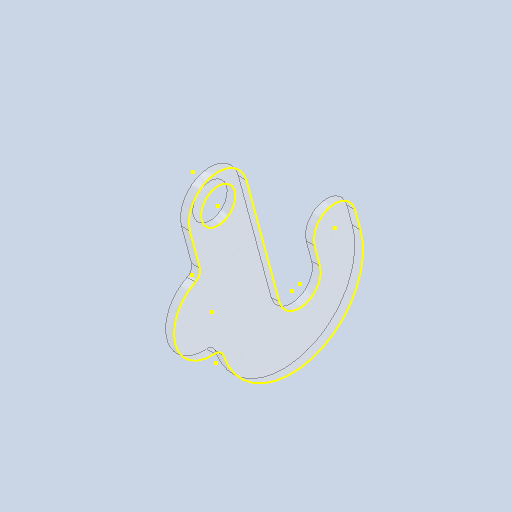
# Autodesk Inventor part: part3
Saved by Autodesk Inventor 2025.2 (Build 292293000, 293)
## iProperties
Created: 2025-02-28
Part Number: part3
Material: アクリル、クリア
Document SubType Name: Modeling
Designer: haruy
Density: 1.19 g/cm^3
Appearance: 透明 - クリア
Author: haruy
Autodesk Inventor part; units mm, degrees
ref_plane "YZ Plane" through (0, 0, 0) normal (1, 0, 0) x (0, 1, 0)
ref_plane "XZ Plane" through (0, 0, 0) normal (0, 1, 0) x (-1, 0, 0)
ref_plane "XY Plane" through (0, 0, 0) normal (0, 0, 1) x (1, 0, 0)
derived "oikon-Sketch-Base.ipt"
sketch "スケッチ1" plane through (100, 0, 0) normal (1, 0, 0) x (0, 1, 0)
  line L0 (0, 0) -> (-50, 0)
  line L1 (-50, 0) -> (-50, -2)
  line L2 (-50, -2) -> (0, -2)
  line L3 (0, -2) -> (0, 0)
  circle A0 centre (-10, -6) radius 4 construction
  circle A1 centre (-10, -6) radius 7
  line L4 (-26, 13) -> (-45, 13)
  line L5 (-45, 13) -> (-45, 2.35)
  line L6 (-45, 2.35) -> (-26, 2.35)
  line L7 (-26, 2.35) -> (-26, 13)
  line L8 (0, 14.6) -> (-50, 14.6)
  line L9 (-50, 14.6) -> (-50, 13)
  line L10 (-50, 13) -> (0, 13)
  line L11 (0, 13) -> (0, 14.6)
  line L12 (0, 36.6) -> (-50, 36.6)
  line L13 (-50, 36.6) -> (-50, 34.6)
  line L14 (-50, 34.6) -> (0, 34.6)
  line L15 (0, 34.6) -> (0, 36.6)
  line L16 (-11.8238, 0.7582) -> (-40.7877, -7.0578)
  arc A2 (-34, 2.35) -> (-32, 2.35) centre (-33, 2.35) ccw
  line L17 (-8.1762, -12.7582) -> (-37.1402, -20.5743)
  line L18 (-40.7877, -7.0578) -> (-37.1402, -20.5743)
  line L19 (-37.1402, -20.5743) -> (-31.9295, -39.8836)
  arc A3 (-37.1402, -20.5743) -> (-34.5348, -30.229) centre (-35.8375, -25.4016) ccw
  line L20 (-34.5348, -30.229) -> (-29.7075, -28.9263)
  line L21 (-29.7075, -28.9263) -> (-28.6397, -32.8834)
  arc A4 (-27.1021, -38.5809) -> (-29.7075, -28.9263) centre (-28.4048, -33.7536) ccw
  line L22 (-27.1021, -38.5809) -> (-31.9295, -39.8836)
  arc A5 (-40.7877, -7.0578) -> (-31.9295, -39.8836) centre (-36.3586, -23.4707) ccw
  line L23 (0, 0) -> (5, 0)
  line L24 (5, 0) -> (5, -2)
  line L25 (5, -2) -> (0, -2)
  line L26 (0, -2) -> (0, 0)
  line L27 (0, 36.6) -> (5, 36.6)
  line L28 (5, 36.6) -> (5, 34.6)
  line L29 (5, 34.6) -> (0, 34.6)
  line L30 (0, 34.6) -> (0, 36.6)
  line L31 (-50, 36.6) -> (-55, 36.6)
  line L32 (-55, 36.6) -> (-55, 34.6)
  line L33 (-55, 34.6) -> (-50, 34.6)
  line L34 (-50, 34.6) -> (-50, 36.6)
  line L35 (-50, 0) -> (-55, 0)
  line L36 (-55, 0) -> (-55, -2)
  line L37 (-55, -2) -> (-50, -2)
  line L38 (-50, -2) -> (-50, 0)
  circle A6 centre (-10, -6) radius 4.1
  arc A7 (-22.4439, -2.1076) -> (-39.8222, -6.7973) centre (-31.133, -4.4525) ccw
  point P0 (-14.1989, 2.35)
  point P1 (-31.9295, -39.8836)
  dimension "d1" = 8.2
  measures "d1" diameter of A6
extrude "押し出し1" add sketch "スケッチ1" along normal blind 2 contours A1 L2 A6 L0 | L0 A1 | A1 L2 L16 L0 | L0 L16 A1 | A1 L2 A6 | A1 L17 L18 L16 L2 | A7 L2 L0 | L0 A7 L6 A2 L7 | A7 L16 L2 | L7 L6 A7 | A3 L19 A5 L18 | L20 A4 L22 L19 | L6 A2 picked at (-34.1225, -4.7033)
fillet "フィレット1" radius 2 2 edges at (101, -22.4439, -2.1076) (101, -39.8222, -6.7973)
sketch "スケッチ2" plane through (102, -37.1402, -20.5743) normal (1, 0, 0) x (0, 0.2605359, -0.9654642)
  arc A0 (-13.9842, -0.7336) -> (20, 0) centre (3, 0) ccw projected
  line L0 (20, 0) -> (20, 5) projected
  arc A1 (20, 5) -> (10, 5) centre (15, 5) ccw projected
  line L1 (10, 5) -> (10, 0) projected
  arc A2 (0, 0) -> (10, 0) centre (5, 0) ccw projected
  line L2 (0, 0) -> (0, 30) projected
  arc A3 (0, 30) -> (-14, 30) centre (-7, 30) ccw projected
  line L3 (-14, 30) -> (-14, 20.8167) projected
  arc A4 (-15.6364, 18.85) -> (-14, 20.8167) centre (-16, 20.8167) ccw projected
  arc A5 (-15.6364, 18.85) -> (-15.6219, 1.1473) centre (-14, 10) ccw projected
  arc A6 (-13.9842, -0.7336) -> (-15.6219, 1.1473) centre (-15.9823, -0.8199) ccw projected
  circle A7 centre (-7, 30) radius 4.1 projected
  point P0 (-10.1874, 41.2179)
